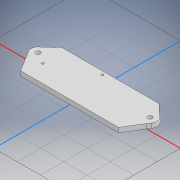
# Autodesk Inventor part: 000.001.012 - Площадка под коммутатор
Saved by Autodesk Inventor 2022 (Build 260153000, 153)
## iProperties
Created: 2023-02-25
Part Number: 000.001.012 - Площадка под коммутатор
Material: Типовые
Document SubType Name: Modeling
Designer: Иван Петров
Density: 1 g/cm^3
Appearance: По умолчанию
Author: Иван Петров
Autodesk Inventor part; units mm, degrees
ref_plane "YZ Plane" through (0, 0, 0) normal (1, 0, 0) x (0, 1, 0)
ref_plane "XZ Plane" through (0, 0, 0) normal (0, 1, 0) x (-1, 0, 0)
ref_plane "XY Plane" through (0, 0, 0) normal (0, 0, 1) x (1, 0, 0)
sketch "Эскиз1" plane through (0, 0, 0) normal (0, 0, 1) x (1, 0, 0)
  point P0 (0, 0)
sketch "Эскиз2" plane through (0, 0, 0) normal (0, 1, 0) x (-1, 0, 0)
  circle A0 centre (38, 0) radius 1
  circle A1 centre (4, -17) radius 1
  line L0 (42, -20) -> (42, 15)
  line L1 (42, 15) -> (35, 15)
  line L2 (35, 15) -> (35, 20)
  line L3 (35, 20) -> (-40, 20)
  line L4 (-40, 20) -> (-40, 15)
  line L5 (-40, 15) -> (-42, 15)
  line L6 (-42, 15) -> (-42, -20)
  line L7 (-42, -20) -> (42, -20)
  line L8 (42, 15) -> (35, 15)
  line L9 (-40, 15) -> (35, 15)
  point P0 (0, 0)
  constraints: 20 end point, 2 centre point, 1 horizontal
extrude "Выдавливание1" add sketch "Эскиз2" along normal blind 4 contours L7 L6 L5 L9 L1 L0
sketch "Эскиз4" plane through (0, 4, 0) normal (0, 1, 0) x (1, 0, 0)
  line L0 (0, 6) -> (-48, 6) construction
  circle A0 centre (-48, 6) radius 2
  circle A1 centre (-48, 6) radius 6
  line L1 (-42, 20) -> (-42, -15) projected
  line L2 (42, 20) -> (-42, 20) projected
  line L3 (-49.2158, 11.8755) -> (-42, 20)
  line L4 (-42, -15) -> (42, -15) projected
  line L5 (-52.5439, 2.0817) -> (-42, -15)
  point P0 (0, 0)
  dimension "d2" = 48
  dimension "d3" = 4
  dimension "d8" = 6
  constraints: 6 end point, 2 centre point, 2 coincident, 2 point on circle, 1 horizontal, 1 tangent, 1 other
  measures "d2" distance of L0.start L0.end
  measures "d3" diameter of A0
  measures "d8" distance from line of L0 point (0, 0)
extrude "Выдавливание2" add sketch "Эскиз4" against normal blind 4
fillet "Сопряжение1" radius 90.25 2 edges at (-52.5439, 2, -2.0817) (-49.2158, 2, -11.8755)
fillet "Сопряжение2" radius 2.5 1 edges at (-42.003, 2, -20)
mirror "Зеркальное отражение1" about plane through (0, 0, 0) normal (1, 0, 0) of "Выдавливание2", "Сопряжение1", "Сопряжение2"
